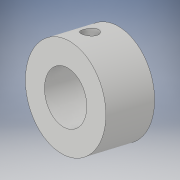
# Autodesk Inventor part: 螺桿固定環
Saved by Autodesk Inventor 2017 (Build 210142000, 142)
## iProperties
Part Number: 螺桿固定環
Material: 一般
Document SubType Name: Modeling
Designer: user
Density: 1 g/cm^3
Appearance: 預設
Author: user
Autodesk Inventor part; units mm, degrees
ref_plane "YZ Plane" through (0, 0, 0) normal (1, 0, 0) x (0, 1, 0)
ref_plane "XZ Plane" through (0, 0, 0) normal (0, 1, 0) x (-1, 0, 0)
ref_plane "XY Plane" through (0, 0, 0) normal (0, 0, 1) x (1, 0, 0)
sketch "草圖1" plane through (0, 0, 0) normal (0, 0, 1) x (1, 0, 0)
  circle A0 centre (0, 0) radius 9.5
  circle A1 centre (0, 0) radius 5
  dimension "d0" = 19
  dimension "d1" = 10
  constraints: 2 centre point, 2 coincident
  measures "d0" diameter of A0
  measures "d1" diameter of A1
extrude "擠出1" add sketch "草圖1" along normal blind 9.66
sketch "草圖2" plane through (0, 0, 0) normal (0, 1, 0) x (-1, 0, 0)
  circle A0 centre (0, 4.83) radius 1.6
  line L0 (-9.5, 0) -> (9.5, 0) projected
  point P0 (0, 0)
  dimension "d4" = 3.2
  dimension "d5" = 6.43
  dimension "d6" = 9.5
  constraints: 1 centre point
  measures "d4" diameter of A0
  measures "d6" horizontal distance of L0.start A0.centre
extrude "擠出2" cut sketch "草圖2" along normal blind 12.5
